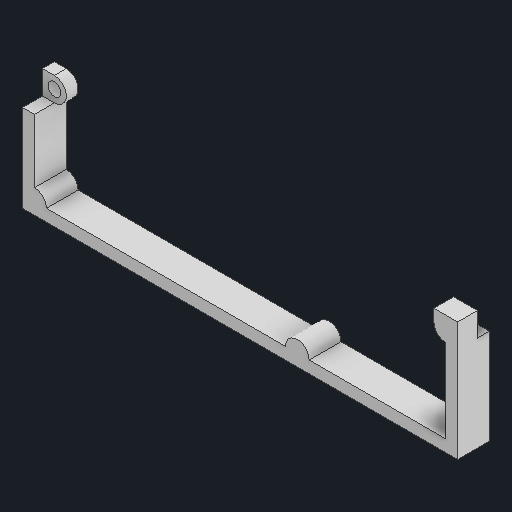
# Autodesk Inventor part: rightwall2
Saved by Autodesk Inventor 2026.2 (Build 302298010, 298A)
## iProperties
Created: 2026-09-07
Part Number: rightwall2
Material: Generic
Document SubType Name: Modeling
Designer: karol
Density: 1 g/cm^3
Appearance: Default
Author: karol
Autodesk Inventor part; units mm, degrees
ref_plane "YZ Plane" through (0, 0, 0) normal (1, 0, 0) x (0, 1, 0)
ref_plane "XZ Plane" through (0, 0, 0) normal (0, 1, 0) x (-1, 0, 0)
ref_plane "XY Plane" through (0, 0, 0) normal (0, 0, 1) x (1, 0, 0)
sketch "Sketch1" plane through (0, 0, 0) normal (0, 0, 1) x (1, 0, 0)
  line L0 (-58, -60) -> (-60, -60) projected
  line L1 (-60, -60) -> (-60, -39.5) projected
  line L2 (-60, -39.5) -> (-58, -39.5) projected
  line L3 (-58, -39.5) -> (-58, -60) projected
  line L4 (49.6, 30) -> (51.6, 30) projected
  line L5 (51.6, 30) -> (51.6, 9.5) projected
  line L6 (51.6, 9.5) -> (49.6, 9.5) projected
  line L7 (49.6, 9.5) -> (49.6, 30) projected
  line L8 (-58, 39.5) -> (-60, 39.5) projected
  line L9 (-60, 39.5) -> (-60, 60) projected
  line L10 (-60, 60) -> (-58, 60) projected
  line L11 (-58, 60) -> (-58, 39.5) projected
  line L12 (-21.6, -39.5) -> (-19.6, -39.5) projected
  line L13 (-19.6, -39.5) -> (-19.6, -60) projected
  line L14 (-19.6, -60) -> (-21.6, -60) projected
  line L15 (-21.6, -60) -> (-21.6, -39.5) projected
  line L16 (51.6, -30) -> (49.6, -30) projected
  line L17 (49.6, -30) -> (49.6, -9.5) projected
  line L18 (49.6, -9.5) -> (51.6, -9.5) projected
  line L19 (51.6, -9.5) -> (51.6, -30) projected
  line L20 (-21.6, 60) -> (-19.6, 60) projected
  line L21 (-19.6, 60) -> (-19.6, 39.5) projected
  line L22 (-19.6, 39.5) -> (-21.6, 39.5) projected
  line L23 (-21.6, 39.5) -> (-21.6, 60) projected
  line L24 (90, -35) -> (90, 35) projected
  line L25 (90, 35) -> (49.6, 35) projected
  line L26 (49.6, 35) -> (49.6, 60) projected
  line L27 (49.6, 60) -> (90, 60) projected
  line L28 (90, 60) -> (90, 90) projected
  line L29 (90, 90) -> (-19.6, 90) projected
  line L30 (-19.6, 90) -> (-19.6, 65) projected
  line L31 (-19.6, 65) -> (-60, 65) projected
  line L32 (-60, 65) -> (-60, 90) projected
  line L33 (-60, 90) -> (-90, 90) projected
  line L34 (-90, 90) -> (-90, -90) projected
  line L35 (-90, -90) -> (-60, -90) projected
  line L36 (-60, -90) -> (-60, -65) projected
  line L37 (-60, -65) -> (-19.6, -65) projected
  line L38 (-19.6, -65) -> (-19.6, -90) projected
  line L39 (-19.6, -90) -> (90, -90) projected
  line L40 (90, -90) -> (90, -60) projected
  line L41 (90, -60) -> (49.6, -60) projected
  line L42 (49.6, -60) -> (49.6, -35) projected
  line L43 (49.6, -35) -> (90, -35) projected
  line L44 (86, -32) -> (73.8, -32) projected
  line L45 (73.8, -32) -> (73.8, -7.5) projected
  line L46 (73.8, -7.5) -> (86, -7.5) projected
  line L47 (86, -7.5) -> (86, -32) projected
  line L48 (65.8, -32) -> (53.6, -32) projected
  line L49 (53.6, -32) -> (53.6, -7.5) projected
  line L50 (53.6, -7.5) -> (65.8, -7.5) projected
  line L51 (65.8, -7.5) -> (65.8, -32) projected
  line L52 (86, -86) -> (70.6, -86) projected
  line L53 (70.6, -86) -> (70.6, -69.8) projected
  line L54 (70.6, -69.8) -> (86, -69.8) projected
  line L55 (86, -69.8) -> (86, -86) projected
  line L56 (86, 86) -> (86, 69.8) projected
  line L57 (86, 69.8) -> (70.6, 69.8) projected
  line L58 (70.6, 69.8) -> (70.6, 86) projected
  line L59 (70.6, 86) -> (86, 86) projected
  line L60 (73.8, 32) -> (86, 32) projected
  line L61 (86, 32) -> (86, 7.5) projected
  line L62 (86, 7.5) -> (73.8, 7.5) projected
  line L63 (73.8, 7.5) -> (73.8, 32) projected
  line L64 (65.8, 32) -> (65.8, 7.5) projected
  line L65 (65.8, 7.5) -> (53.6, 7.5) projected
  line L66 (53.6, 7.5) -> (53.6, 32) projected
  line L67 (53.6, 32) -> (65.8, 32) projected
  line L68 (-69.6, -87) -> (-85, -87) projected
  line L69 (-85, -87) -> (-85, -70.8) projected
  line L70 (-85, -70.8) -> (-69.6, -70.8) projected
  line L71 (-69.6, -70.8) -> (-69.6, -87) projected
  line L72 (-56, -62) -> (-56, -37.5) projected
  line L73 (-56, -37.5) -> (-43.8, -37.5) projected
  line L74 (-43.8, -37.5) -> (-43.8, -62) projected
  line L75 (-43.8, -62) -> (-56, -62) projected
  line L76 (-56, 62) -> (-43.8, 62) projected
  line L77 (-43.8, 62) -> (-43.8, 37.5) projected
  line L78 (-43.8, 37.5) -> (-56, 37.5) projected
  line L79 (-56, 37.5) -> (-56, 62) projected
  line L80 (-23.6, 62) -> (-23.6, 37.5) projected
  line L81 (-23.6, 37.5) -> (-35.8, 37.5) projected
  line L82 (-35.8, 37.5) -> (-35.8, 62) projected
  line L83 (-35.8, 62) -> (-23.6, 62) projected
  line L84 (-23.6, -62) -> (-35.8, -62) projected
  line L85 (-35.8, -62) -> (-35.8, -37.5) projected
  line L86 (-35.8, -37.5) -> (-23.6, -37.5) projected
  line L87 (-23.6, -37.5) -> (-23.6, -62) projected
  line L88 (-85, 87) -> (-69.6, 87) projected
  line L89 (-69.6, 87) -> (-69.6, 70.8) projected
  line L90 (-69.6, 70.8) -> (-85, 70.8) projected
  line L91 (-85, 70.8) -> (-85, 87) projected
  circle A0 centre (87, -63) radius 2 projected
  line L92 (90, -60) -> (90, -66) projected
  line L93 (84, -60) -> (90, -60) projected
  line L94 (84, -63) -> (84, -60) projected
  line L95 (90, -66) -> (87, -66) projected
  line L96 (-19.6, 68) -> (-16.6, 68) projected
  line L97 (-16.6, 68) -> (-16.6, 84) projected
  line L98 (-13.6, 87) -> (46.6, 87) projected
  line L99 (52.6, 87) -> (87, 87) projected
  line L100 (87, 87) -> (87, 66) projected
  line L101 (84, 63) -> (84, 60) projected
  line L102 (84, 60) -> (90, 60) projected
  line L103 (90, 60) -> (90, 90) projected
  line L104 (90, 90) -> (-19.6, 90) projected
  line L105 (-19.6, 90) -> (-19.6, 68) projected
  line L106 (90, -66) -> (87, -66)
  line L107 (87, -66) -> (87, -90)
  line L108 (87, -90) -> (90, -90)
  line L109 (90, -90) -> (90, -66)
  line L110 (87, -90) -> (-19.6, -90)
  line L111 (-19.6, -90) -> (-19.6, -87)
  line L112 (-19.6, -87) -> (87, -87)
  line L113 (87, -87) -> (87, -90)
  line L114 (-19.6, -87) -> (-16.6, -87)
  line L115 (-16.6, -87) -> (-16.6, -65)
  line L116 (-16.6, -65) -> (-19.6, -65)
  line L117 (-19.6, -65) -> (-19.6, -87)
  line L118 (-19.6, -65) -> (-16.6, -65)
  line L119 (-16.6, -65) -> (-16.6, -68)
  line L120 (-16.6, -68) -> (-19.6, -68)
  line L121 (-19.6, -68) -> (-19.6, -65)
  line L122 (-19.6, -68) -> (-13.6, -68)
  line L123 (-13.6, -68) -> (-13.6, -62)
  line L124 (-13.6, -62) -> (-19.6, -62)
  line L125 (-19.6, -62) -> (-19.6, -68)
  line L126 (-19.6, -90) -> (-13.6, -90)
  line L127 (-13.6, -90) -> (-13.6, -84)
  line L128 (-13.6, -84) -> (-19.6, -84)
  line L129 (-19.6, -84) -> (-19.6, -90)
  line L130 (46.6, -90) -> (52.6, -90)
  line L131 (52.6, -90) -> (52.6, -84)
  line L132 (52.6, -84) -> (46.6, -84)
  line L133 (46.6, -84) -> (46.6, -90)
  circle A1 centre (-63, -65) radius 1.5 projected
  circle A2 centre (-16.6, -87) radius 1.5 projected
  circle A3 centre (49.6, -87) radius 1.5 projected
  circle A4 centre (46.6, -60) radius 1.5 projected
  circle A5 centre (87, -63) radius 1.5 projected
  circle A6 centre (46.6, -32) radius 1.5 projected
  circle A7 centre (46.6, 32) radius 1.5 projected
  circle A8 centre (87, 63) radius 1.5 projected
  circle A9 centre (46.6, 60) radius 1.5 projected
  circle A10 centre (49.6, 87) radius 1.5 projected
  circle A11 centre (-16.6, 87) radius 1.5 projected
  circle A12 centre (-16.6, 65) radius 1.5 projected
  circle A13 centre (-63, 65) radius 1.5 projected
  arc A14 (87, 66) -> (84, 63) centre (87, 63) ccw projected
  arc A15 (-16.6, 84) -> (-13.6, 87) centre (-16.6, 87) ccw projected
  arc A16 (46.6, 87) -> (52.6, 87) centre (49.6, 87) ccw projected
  arc A17 (84, -63) -> (87, -66) centre (87, -63) ccw projected
  line L134 (-76, -39.25) -> (-82, -39.25) projected
  line L135 (-82, -39.25) -> (-82, -20.75) projected
  line L136 (-82, -20.75) -> (-76, -20.75) projected
  line L137 (-76, -20.75) -> (-76, -39.25) projected
  line L138 (-76, 20.75) -> (-82, 20.75) projected
  line L139 (-82, 20.75) -> (-82, 39.25) projected
  line L140 (-82, 39.25) -> (-76, 39.25) projected
  line L141 (-76, 39.25) -> (-76, 20.75) projected
  circle A18 centre (-87, 55.8) radius 1.25 projected
  circle A19 centre (-87, -55.8) radius 1.25 projected
  point P0 (0, 0)
  point P1 (52.6, -87)
  point P2 (46.6, -87)
  point P3 (-13.6, -87)
  point P4 (-16.6, -84)
  dimension "d0" = 3
  dimension "d1" = 3
  dimension "d2" = 6
  dimension "d3" = 6
  dimension "d4" = 6
  dimension "d5" = 6
  dimension "d6" = 6
  dimension "d7" = 6
  constraints: 56 end point, 14 parallel, 7 horizontal, 7 perpendicular, 4 point on line
  measures "d0" distance of L116.end L115.end
  measures "d1" distance of L118.end L119.end
  measures "d2" distance of L124.end L123.end
  measures "d3" distance of L123.end L122.end
  measures "d4" distance of L128.end L127.end
  measures "d5" distance of L127.end L126.end
  measures "d6" distance of L132.end L131.end
  measures "d7" distance of L131.end L130.end
extrude "Extrusion1" add sketch "Sketch1" along normal blind 8 contours L41 L40 L95 A17 L94 | L40 L39 L107 L95 | L107 L39 L131 L112 | L131 L39 L133 L112 A3 | L112 A3 L133 L132 L131 | A3 L112 | L112 A3 | L39 L127 L112 L133 | L39 L38 L112 A2 L127 | L112 A2 L115 L128 L127 | L38 L128 L115 A2 L112 | A2 L112 | L112 L115 A2 | L38 L120 L115 L128 | A2 L115 L112 | L38 L116 L115 L120 | L115 L116 L125 L124 L123 L122 | A0 | A5
sketch "Sketch2" plane through (0, 0, 0) normal (0, 0, -1) x (-1, 0, 0)
  line L0 (-84, -66) -> (-87, -66) projected
  line L1 (-90, -90) -> (-90, -60) projected
  line L2 (-84, -66) -> (-90, -66)
  line L3 (-90, -66) -> (-90, -60)
  line L4 (-90, -60) -> (-84, -60)
  line L5 (-84, -60) -> (-84, -66)
  line L6 (-84, -60) -> (-90, -66)
  line L7 (-90, -60) -> (-84, -66)
  circle A0 centre (-87, -63) radius 2
  line L8 (-52.6, -84) -> (-46.6, -84) projected
  line L9 (-46.6, -84) -> (-52.6, -90)
  line L10 (19.6, -90) -> (-90, -90) projected
  line L11 (-52.6, -84) -> (-46.6, -90)
  line L12 (-46.6, -90) -> (-46.6, -84)
  line L13 (-52.6, -84) -> (-52.6, -90)
  circle A1 centre (-49.6, -87) radius 2
  line L14 (13.6, -84) -> (16.6, -84) projected
  line L15 (13.6, -84) -> (19.6, -90)
  line L16 (19.6, -62) -> (19.6, -90) projected
  line L17 (19.6, -84) -> (13.6, -90)
  line L18 (19.6, -84) -> (13.6, -84)
  circle A2 centre (16.6, -87) radius 2
  line L19 (13.6, -68) -> (13.6, -62) projected
  line L20 (13.6, -68) -> (19.6, -62)
  line L21 (19.6, -68) -> (13.6, -62)
  line L22 (13.6, -62) -> (13.6, -68)
  line L23 (19.6, -68) -> (13.6, -68)
  circle A3 centre (16.6, -65) radius 2
  point P0 (0, 0)
  point P1 (19.6, -87)
  dimension "d10" = 4
  dimension "d11" = 4
  dimension "d12" = 4
  dimension "d13" = 4
  constraints: 34 end point, 6 perpendicular, 4 centre point, 4 midpoint, 4 point on line, 3 parallel, 2 collinear, 1 horizontal, 1 vertical
  measures "d10" diameter of A0
  measures "d11" diameter of A1
  measures "d12" diameter of A2
  measures "d13" diameter of A3
extrude "Extrusion2" cut sketch "Sketch2" against normal blind 6 contours A1 L9 L11 | L11 L9 A1 | A1 L11 L9 | L11 A1 L9 | A2 L17 L15 | L15 L17 A2 | A2 L15 L17 | L15 A2 L17
extrude "Extrusion3" cut sketch "Sketch2" against normal blind 7 contours A0 L6 L7 | L7 L6 A0 | L6 L7 A0 | L6 A0 L7
extrude "Extrusion4" cut sketch "Sketch2" against normal blind 3 contours L7 A0 L6 L5 | L0 L2 L6 A0 L7 | L6 A0 L7 L4 | L1 L7 A0 L6
sketch "Sketch3" plane through (0, 0, 8) normal (0, 0, 1) x (1, 0, 0)
  line L0 (-16.6, -68) -> (-13.6, -68) projected
  line L1 (-19.6, -62) -> (-19.6, -90) projected
  line L2 (-13.6, -68) -> (-19.6, -62)
  line L3 (-19.6, -62) -> (-13.6, -62)
  line L4 (-13.6, -62) -> (-19.6, -68)
  line L5 (-13.6, -68) -> (-19.6, -68)
  line L6 (-13.6, -62) -> (-13.6, -68)
  circle A0 centre (-16.6, -65) radius 1.65
  point P0 (0, 0)
  point P1 (-19.6, -87)
  point P2 (-17.7667, -66.1667)
  point P3 (-17.7667, -63.8333)
  dimension "d20" = 3.3
  constraints: 10 end point, 3 perpendicular, 1 centre point, 1 horizontal, 1 midpoint, 1 point on line
  measures "d20" diameter of A0
extrude "Extrusion5" cut sketch "Sketch3" against normal blind 5 contours L5 L4 A0 L2 L0 | L2 A0 L4 L6 | L1 L2 A0 L4 | L4 A0 L2 L3
extrude "Extrusion6" cut sketch "Sketch3" against normal blind 8 contours A0 L4 L2 | L2 L4 A0 | A0 L2 L4 | L2 A0 L4
fillet "Fillet1" radius 3 5 edges at (52.6, -84, 4) (46.6, -84, 4) (-13.6, -68, 1.5) (-13.6, -62, 1.5) (-13.6, -84, 4)
body "Solid1"
